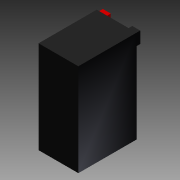
# Autodesk Inventor part: TB1272-Battery
Saved by Autodesk Inventor 2012 (Build 160160000, 160)
## iProperties
Created: 2013-07-14
Part Number: TB1272-Battery
Material: Default
Document SubType Name: Modeling
Designer: joe_000
Density: 1 g/cm^3
Author: joe_000
Autodesk Inventor part; units mm, degrees
ref_plane "YZ Plane" through (0, 0, 0) normal (1, 0, 0) x (0, 1, 0)
ref_plane "XZ Plane" through (0, 0, 0) normal (0, 1, 0) x (-1, 0, 0)
ref_plane "XY Plane" through (0, 0, 0) normal (0, 0, 1) x (1, 0, 0)
sketch "Sketch1" plane through (0, 0, 0) normal (0, 0, 1) x (1, 0, 0)
  line L0 (0, 0) -> (65, 0)
  line L1 (65, 0) -> (65, 95)
  line L2 (65, 95) -> (0, 95)
  line L3 (0, 95) -> (0, 0)
  dimension "d0" = 95
  dimension "d1" = 65
  constraints: 8 end point, 2 parallel, 1 horizontal, 1 perpendicular
  measures "d0" distance of L0.end L1.end
  measures "d1" distance of L1.end L2.end
extrude "Extrusion1" add sketch "Sketch1" along normal blind 151
sketch "Sketch2" plane through (0, 95, 0) normal (0, 1, 0) x (1, 0, 0)
  line L0 (2, -149) -> (15, -149)
  line L1 (15, -149) -> (15, -130)
  line L2 (15, -130) -> (2, -130)
  line L3 (2, -130) -> (2, -149)
  line L4 (0, -151) -> (65, -151) projected
  line L5 (0, 0) -> (0, -151) projected
  dimension "d6" = 2
  dimension "d7" = 19
  dimension "d8" = 13
  dimension "d9" = 2
  constraints: 8 end point, 2 parallel, 1 horizontal, 1 perpendicular
  measures "d6" distance between parallel lines of L5 L3
  measures "d7" distance of L2.end L0.start
  measures "d8" distance of L1.end L2.end
  measures "d9" distance between parallel lines of L4 L0
extrude "Extrusion2" add sketch "Sketch2" along normal blind 8 separate body
sketch "Sketch3" plane through (0, 95, 0) normal (0, 1, 0) x (1, 0, 0)
  line L0 (0, -151) -> (65, -151) projected
  line L1 (65, 0) -> (65, -151) projected
  line L2 (63, -149) -> (50, -149)
  line L3 (50, -149) -> (50, -130)
  line L4 (50, -130) -> (63, -130)
  line L5 (63, -130) -> (63, -149)
  dimension "d10" = 19
  dimension "d11" = 13
  dimension "d12" = 2
  dimension "d13" = 2
  constraints: 8 end point, 2 parallel, 1 horizontal, 1 perpendicular
  measures "d10" distance of L4.end L2.start
  measures "d11" distance of L2.start L2.end
  measures "d12" distance between parallel lines of L0 L2
  measures "d13" distance between parallel lines of L1 L5
extrude "Extrusion3" add sketch "Sketch3" along normal blind 8 separate body
body "Solid1"
body "Solid2"
body "Solid3"
